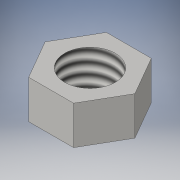
# Autodesk Inventor part: nut
Saved by Autodesk Inventor 2016 (Build 200138000, 138)
## iProperties
Created: 2015-05-13
Part Number: nut
Material: Generic
Document SubType Name: Modeling
Designer: Admin
Density: 1 g/cm^3
Appearance: Default
Author: Admin
Autodesk Inventor part; units mm, degrees
ref_plane "YZ Plane" through (0, 0, 0) normal (1, 0, 0) x (0, 1, 0)
ref_plane "XZ Plane" through (0, 0, 0) normal (0, 1, 0) x (-1, 0, 0)
ref_plane "XY Plane" through (0, 0, 0) normal (0, 0, 1) x (1, 0, 0)
sketch "Sketch1" plane through (0, 0, 0) normal (0, 1, 0) x (-1, 0, 0)
  line L0 (6.6675, -3.8495) -> (8.89, 0)
  line L1 (6.6675, -3.8495) -> (2.2225, -3.8495)
  line L2 (2.2225, -3.8495) -> (0, 0)
  line L3 (6.6675, 3.8495) -> (8.89, 0)
  line L4 (6.6675, 3.8495) -> (2.2225, 3.8495)
  line L5 (2.2225, 3.8495) -> (0, 0)
  circle A0 centre (4.445, 0) radius 2.5019
  dimension "d5" = 5.0038
  constraints: 12 end point, 1 centre point
  measures "d5" diameter of A0
extrude "Extrusion1" add sketch "Sketch1" along normal blind 3.81
thread "Thread1" size "12-24 UNC" class "2B" standard "ANSI Unified Screw Threads" full length
body "Solid1"
